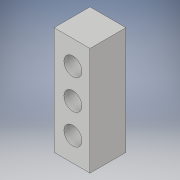
# Autodesk Inventor part: traffic light
Saved by Autodesk Inventor 2019 (Build 230136000, 136)
## iProperties
Created: 2022-02-22
Part Number: traffic light
Material: Generic
Document SubType Name: Modeling
Designer: BoboPC
Density: 1 g/cm^3
Appearance: Default
Author: BoboPC
Autodesk Inventor part; units mm, degrees
ref_plane "YZ Plane" through (0, 0, 0) normal (1, 0, 0) x (0, 1, 0)
ref_plane "XZ Plane" through (0, 0, 0) normal (0, 1, 0) x (-1, 0, 0)
ref_plane "XY Plane" through (0, 0, 0) normal (0, 0, 1) x (1, 0, 0)
sketch "Sketch1" plane through (0, 0, 0) normal (0, 0, 1) x (1, 0, 0)
  line L0 (0, 0) -> (304.8, 0)
  line L1 (304.8, 0) -> (304.8, 914.4)
  line L2 (304.8, 914.4) -> (0, 914.4)
  line L3 (0, 914.4) -> (0, 0)
  dimension "d0" = 304.8
  dimension "d1" = 914.4
  constraints: 8 end point, 2 parallel, 1 horizontal, 1 perpendicular
  measures "d0" distance of L2.end L1.end
  measures "d1" distance of L1.end L0.end
extrude "Extrusion1" add sketch "Sketch1" along normal blind 304.8
sketch "Sketch2" plane through (0, 0, 304.8) normal (0, 0, 1) x (1, 0, 0)
  line L0 (0, 0) -> (304.8, 0) projected
  line L1 (304.8, 0) -> (304.8, 914.4) projected
  line L2 (304.8, 914.4) -> (0, 914.4) projected
  line L3 (0, 914.4) -> (0, 0) projected
  circle A0 centre (160.2433, 711.2) radius 76.2
  circle A1 centre (160.2433, 457.2) radius 76.2
  circle A2 centre (160.2433, 203.2) radius 76.2
  line L4 (304.8, 914.4) -> (0, 914.4) construction
  line L5 (160.2433, 914.4) -> (160.2433, 895.9675) construction
  dimension "d4" = 152.4
  dimension "d5" = 0
  dimension "d6" = 152.4
  dimension "d7" = 152.4
  dimension "d8" = 254
  dimension "d9" = 254
  dimension "d10" = -203.2
  constraints: 3 centre point, 2 end point, 2 vertical alignment, 1 point on line, 1 vertical
  measures "d4" diameter of A0
  measures "d5" distance from line of L5 A0.centre
  measures "d6" diameter of A1
  measures "d7" diameter of A2
  measures "d8" distance of A1.centre A0.centre
  measures "d9" distance of A2.centre A1.centre
  measures "d10" distance from line of L0 A2.centre
extrude "Extrusion2" cut sketch "Sketch2" against normal blind 152.4 contours A0 | A1 | A2
equation "\"d6\" = d4"
equation "\"d7\" = d4"
equation "\"d9\" = d8"
equation "\"d10\" = -0.5 * d1 + d8"
body "Solid1"
